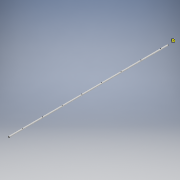
# Autodesk Inventor part: water out put
Saved by Autodesk Inventor 2017 (Build 210142000, 142)
## iProperties
Created: 2017-11-09
Part Number: water out put
Material: Generic
Document SubType Name: Modeling
Designer: DesignPC02
Density: 1 g/cm^3
Appearance: Default
Author: DesignPC02
Autodesk Inventor part; units mm, degrees
ref_plane "YZ Plane" through (0, 0, 0) normal (1, 0, 0) x (0, 1, 0)
ref_plane "XZ Plane" through (0, 0, 0) normal (0, 1, 0) x (-1, 0, 0)
ref_plane "XY Plane" through (0, 0, 0) normal (0, 0, 1) x (1, 0, 0)
sketch "Sketch2" plane through (0, 0, 0) normal (0, 1, 0) x (-1, 0, 0)
  circle A0 centre (0, 0) radius 11
  circle A1 centre (0, 0) radius 10
  dimension "d0" = 22
  dimension "d1" = 1
  constraints: 2 centre point, 1 coincident
  measures "d0" diameter of A0
  measures "d1" radial gap between concentric circles of A0 A1
extrude "Extrusion1" add sketch "Sketch2" along normal mid plane 2750
sketch "Sketch4" plane through (0, 0, 0) normal (0, 0, 1) x (1, 0, 0)
  line L0 (-11, -1375) -> (11, -1375) projected
  circle A0 centre (0, -1135) radius 4
  line L1 (0, -1375) -> (0, -1288.6892)
  circle A1 centre (0, -795) radius 4
  circle A2 centre (0, -455) radius 4
  circle A3 centre (0, -115) radius 4
  circle A4 centre (0, 225) radius 4
  circle A5 centre (0, 565) radius 4
  circle A6 centre (0, 905) radius 4
  circle A7 centre (0, 1245) radius 4
  point P0 (0, 0)
  dimension "d10" = 8
  dimension "d11" = 240
  dimension "d26" = 8
  dimension "d27" = 340
  dimension "d30" = 340
  constraints: 8 centre point, 2 end point, 2 vertical, 1 midpoint, 12 other
  measures "d10" diameter of A0
  measures "d11" distance from line of L0 A0.centre
  measures "d26" diameter of A1
  measures "d27" distance of A0.centre A1.centre
  measures "d30" distance of A1.centre A2.centre
extrude "Extrusion2" cut sketch "Sketch4" along normal through all
body "Solid1"
